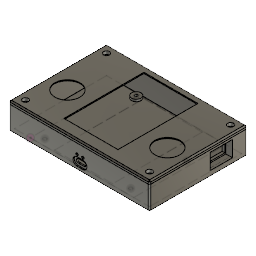
Control-Case (Autodesk Fusion 360 design; units mm, degrees)
Autodesk Fusion 360 part; units mm, degrees
sketch "Skizze1" plane through (0, 0, 0) normal (0, 0, 1) x (1, 0, 0) in component "Case-Bottom"
  line L0 (0, 0) -> (99, 0) construction
  line L1 (99, 0) -> (99, 88) construction
  line L2 (99, 88) -> (0, 88) construction
  line L3 (0, 88) -> (0, 0) construction
  circle A0 centre (7.8, 6.1) radius 1.5 construction
  circle A1 centre (90, 6.1) radius 1.5 construction
  circle A2 centre (94, 55.7) radius 1.5 construction
  circle A3 centre (17.6, 83.8) radius 1.5 construction
  line L4 (21.8, 86.9) -> (77.5, 86.9) construction
  line L5 (77.5, 86.9) -> (77.5, 1.4) construction
  line L6 (77.5, 1.4) -> (21.8, 1.4) construction
  line L7 (21.8, 1.4) -> (21.8, 86.9) construction
  line L8 (-15.1, 0) -> (114.1, 0) construction
  line L9 (114.1, 0) -> (114.1, 88) construction
  line L10 (114.1, 88) -> (-15.1, 88) construction
  line L11 (-15.1, 88) -> (-15.1, 0) construction
  dimension "d1" = 99
  dimension "d2" = 88
  dimension "d3" = 3
  dimension "d4" = 1.4
  dimension "d5" = 86.9
  dimension "d6" = 21.8
  dimension "d7" = 77.5
  dimension "d8" = 7.8
  dimension "d9" = 6.1
  dimension "d10" = 83.8
  dimension "d11" = 17.6
  dimension "d12" = 94
  dimension "d13" = 55.7
  dimension "d14" = 6.1
  dimension "d15" = 90
  dimension "d16" = 15.1
  dimension "d17" = 15.1
  constraint horizontal L0
  constraint vertical L1
  constraint horizontal L2
  constraint vertical L3
  constraint coincident L0.start L3.end
  constraint equal A0 A1
  constraint equal A1 A2
  constraint equal A2 A3
  constraint horizontal L4
  constraint vertical L5
  constraint horizontal L6
  constraint vertical L7
  constraint horizontal L8
  constraint vertical L9
  constraint horizontal L10
  constraint vertical L11
  constraint collinear L2 L10
  constraint collinear L0 L8
  measures "d1" distance of L0.start L0.end
  measures "d2" distance of L0.start L2.end
  measures "d3" diameter of A0
  measures "d4" distance of L0 L6
  measures "d5" distance of L0 L4
  measures "d6" distance of L3 L7
  measures "d7" distance of L3 L5
  measures "d8" distance of L3 A0.centre
  measures "d9" distance of L0 A0.centre
  measures "d10" distance of L0 A3.centre
  measures "d11" distance of L3 A3.centre
  measures "d12" distance of L3 A2.centre
  measures "d13" distance of L0 A2.centre
  measures "d14" distance of L0 A1.centre
  measures "d15" distance of L3 A1.centre
  measures "d16" distance of L3 L11
  measures "d17" distance of L1 L9
sketch "Skizze2" plane through (0, 0, 0) normal (0, 0, 1) x (1, 0, 0) in component "Case-Bottom"
  line L0 (114.1, 0) -> (114.1, 88)
  line L1 (114.1, 88) -> (-15.1, 88)
  line L2 (-15.1, 0) -> (114.1, 0)
  line L3 (-15.1, 88) -> (-15.1, 0)
  line L4 (-15.4, -0.3) -> (114.4, -0.3)
  line L5 (114.4, -0.3) -> (114.4, 88.3)
  line L6 (114.4, 88.3) -> (-15.4, 88.3)
  line L7 (-15.4, 88.3) -> (-15.4, -0.3)
  line L8 (-17.9, 90.8) -> (-17.9, -2.8)
  line L9 (-17.9, -2.8) -> (116.9, -2.8)
  line L10 (116.9, -2.8) -> (116.9, 90.8)
  line L11 (116.9, 90.8) -> (-17.9, 90.8)
  dimension "d18" = 0.3
  dimension "d19" = 2.8
extrude "Extrusion1" add sketch "Skizze2" against normal blind 2 contours L0 L1 L2 L3 | L4 L5 L6 L7 | L8 L9 L10 L11 makes body 1 in component "Case-Bottom"
sketch "Skizze3" plane through (0, 0, 0) normal (0, 0, 1) x (-1, 0, 0) in component "Case-Bottom"
  line L0 (-116.9, -90.8) -> (17.9, -90.8)
  line L1 (17.9, -90.8) -> (17.9, 2.8)
  line L2 (17.9, 2.8) -> (-116.9, 2.8)
  line L3 (-116.9, 2.8) -> (-116.9, -90.8)
  circle A0 centre (-7.8, -6.1) radius 1.5
  circle A1 centre (-17.6, -83.8) radius 1.5
  circle A2 centre (-94, -55.7) radius 1.5
  circle A3 centre (-90, -6.1) radius 1.5
  circle A4 centre (-7.8, -6.1) radius 4.5
  circle A5 centre (-90, -6.1) radius 4.5
  circle A6 centre (-94, -55.7) radius 4.5
  circle A7 centre (-17.6, -83.8) radius 4.5
  circle A8 centre (-7.8, -6.1) radius 1.35
  circle A9 centre (-17.6, -83.8) radius 1.35
  circle A10 centre (-94, -55.7) radius 1.35
  circle A11 centre (-90, -6.1) radius 1.35
  dimension "d22" = 3
  dimension "d23" = 3
  dimension "d25" = 3
  dimension "d26" = 3
  dimension "d113" = 2.7
  constraint concentric A0 A8
  constraint concentric A1 A9
  constraint concentric A2 A10
  constraint concentric A3 A11
  constraint equal A10 A11
  constraint equal A9 A10
  constraint equal A8 A9
  measures "d22" distance of A0
  measures "d23" distance of A3
  measures "d25" distance of A2
  measures "d26" distance of A1
  measures "d113" diameter of A8
extrude "Extrusion2" add sketch "Skizze3" along normal blind 2 contours A0 | A1 | A2 | A3 | A4 | A5 | A6 | A7 bodies 1 in component "Case-Bottom"
extrude "Extrusion3" cut 4 faces at (93.7048, 56.1487, 0) (7.6775, 6.2407, 0) (89.3906, 5.7482, 0) (18.3106, 84.193, 0) along direction (0, 0, -1) blind 1 on bodies 1 bodies 1 in component "Case-Bottom"
sketch "Skizze4" plane through (0, 0, 0) normal (0, 0, 1) x (-1, 0, 0) in component "Case-Bottom"
  circle A0 centre (-17.6, -83.8) radius 4.5
  circle A1 centre (-94, -55.7) radius 4.5
  line L0 (-116.9, -90.8) -> (17.9, -90.8)
  line L1 (17.9, -90.8) -> (17.9, 2.8)
  line L2 (17.9, 2.8) -> (-116.9, 2.8)
  line L3 (-116.9, 2.8) -> (-116.9, -90.8)
  circle A2 centre (-7.8, -6.1) radius 4.5
  circle A3 centre (-90, -6.1) radius 4.5
  line L4 (15.4, -88.3) -> (15.4, 0.3)
  line L5 (15.4, 0.3) -> (-114.4, 0.3)
  line L6 (-114.4, 0.3) -> (-114.4, -88.3)
  line L7 (-114.4, -88.3) -> (15.4, -88.3)
  dimension "d31" = -2.5
extrude "Extrusion4" add sketch "Skizze4" along normal blind 20.8 separate body contours L0 L1 L2 L3 makes body 2 in component "Case-Bottom"
combine "Kombinieren1" operation add target body 1 tool bodies 2 in component "Case-Bottom"
sketch "Skizze1 (2)" plane through (0, 0, 20.8) normal (0, 0, 1) x (-1, 0, 0) in component "Case-Top"
  line L0 (15.4, -88.3) -> (-114.4, -88.3)
  line L1 (-114.4, -88.3) -> (-114.4, 0.3)
  line L2 (15.4, 0.3) -> (15.4, -88.3)
  line L3 (-116.9, 2.8) -> (-116.9, -90.8)
  line L4 (-116.9, -90.8) -> (17.9, -90.8)
  line L5 (17.9, -90.8) -> (17.9, 2.8)
  line L6 (17.9, 2.8) -> (-116.9, 2.8)
  line L7 (17.9, 2.8) -> (-116.9, 2.8)
  line L8 (-116.9, 2.8) -> (-116.9, -90.8)
  line L9 (-116.9, -90.8) -> (17.9, -90.8)
  line L10 (17.9, -90.8) -> (17.9, 2.8)
  line L11 (-21.8, -1.4) -> (-21.8, -86.9)
  line L12 (-77.5, -1.4) -> (-21.8, -1.4)
  line L13 (-77.5, -86.9) -> (-77.5, -1.4)
  line L14 (-21.8, -86.9) -> (-77.5, -86.9)
  line L15 (-23.8, -84.9) -> (-75.5, -84.9)
  line L16 (-75.5, -84.9) -> (-75.5, -8.4)
  line L17 (-75.5, -8.4) -> (-23.8, -8.4)
  line L18 (-23.8, -8.4) -> (-23.8, -84.9)
  circle A0 centre (-1.8, -33.7) radius 12
  circle A1 centre (-97.5, -33.7) radius 12
  line L19 (-114.4, 0.3) -> (15.4, 0.3)
  line L20 (-21.6, -1.2) -> (-21.6, -87.1)
  line L21 (-21.6, -87.1) -> (-77.7, -87.1)
  line L22 (-77.7, -87.1) -> (-77.7, -1.2)
  line L23 (-77.7, -1.2) -> (-21.6, -1.2)
  dimension "d34" = 7
  dimension "d35" = 2
  dimension "d36" = 2
  dimension "d37" = 2
  dimension "d43" = 34
  dimension "d44" = 34
  dimension "d45" = 24
  dimension "d46" = 20
  dimension "d47" = 20
  dimension "d112" = -0.2
  constraint horizontal L7
  constraint vertical L8
  constraint horizontal L9
  constraint vertical L10
  constraint coincident L3.end L4.start
  constraint coincident L5.end L6.start
  constraint horizontal L15
  constraint vertical L16
  constraint horizontal L17
  constraint vertical L18
  constraint equal A0 A1
  measures "d34" distance of L12 L17
  measures "d35" distance of L13 L16
  measures "d36" distance of L14 L15
  measures "d37" distance of L11 L18
  measures "d43" distance of A0.centre L19
  measures "d44" distance of A1.centre L19
  measures "d45" diameter of A0
  measures "d46" distance of L11 A0.centre
  measures "d47" distance of L13 A1.centre
extrude "Extrusion1'" add sketch "Skizze1 (2)" along normal blind 2 separate body contours L0 L1 L2 L19 | L3 L4 L5 L6 L7 L8 L9 L10 | L11 L12 L13 L14 | L20 L21 L22 L23 makes body 3 in component "Case-Top"
extrude "Extrusion2'" cut sketch "Skizze1 (2)" along normal blind 1 contours L11 L12 L13 L14 | L20 L21 L22 L23 bodies 3 in component "Case-Top"
chamfer "Fase1" distance 1.4 angle 45 2 edges at (12.9879, 29.3606, 20.8) (108.6879, 29.3606, 20.8) on bodies 3 in component "Case-Top"
sketch "Skizze2 (2)" plane through (0, 0, 22.8) normal (0, 0, 1) x (-1, 0, 0) in component "Case-Top"
  line L0 (-75.5, -8.4) -> (-23.8, -8.4)
  line L1 (-23.8, -8.4) -> (-23.8, -84.9)
  line L2 (-23.8, -84.9) -> (-75.5, -84.9)
  line L3 (-75.5, -84.9) -> (-75.5, -8.4)
  circle A0 centre (-97.5, -33.7) radius 12
  circle A1 centre (-1.8, -33.7) radius 12
  line L4 (17.9, -90.8) -> (17.9, 2.8)
  line L5 (17.9, 2.8) -> (-116.9, 2.8)
  line L6 (-116.9, 2.8) -> (-116.9, -90.8)
  line L7 (-116.9, -90.8) -> (17.9, -90.8)
  line L8 (-108.9, -82.8) -> (9.9, -82.8) construction
  line L9 (9.9, -82.8) -> (9.9, -5.2) construction
  line L10 (9.9, -5.2) -> (-108.9, -5.2) construction
  line L11 (-108.9, -5.2) -> (-108.9, -82.8) construction
  circle A2 centre (9.9, -5.2) radius 2.8
  circle A3 centre (9.9, -82.8) radius 2.8
  circle A4 centre (-108.9, -82.8) radius 2.8
  circle A5 centre (-108.9, -5.2) radius 2.8
  dimension "d49" = -8
  dimension "d50" = 5.6
  constraint coincident L9.end L10.start
  constraint coincident L8.end L9.start
  constraint coincident L8.start L11.end
  constraint coincident L10.end L11.start
  constraint equal A4 A5
  constraint equal A3 A4
  constraint equal A2 A3
  measures "d50" diameter of A2
extrude "Extrusion3'" cut sketch "Skizze2 (2)" against normal blind 2 contours A2 | A3 | A4 | A5 bodies 3 in component "Case-Top"
sketch "Skizze3 (2)" plane through (0, 0, 20.8) normal (0, 0, -1) x (1, 0, 0) in component "Case-Top"
  circle A0 centre (108.9, -82.8) radius 2.8
  circle A1 centre (108.9, -5.2) radius 2.8
  circle A2 centre (-9.9, -82.8) radius 2.8
  circle A3 centre (-9.9, -5.2) radius 2.8
  circle A4 centre (1.8, -33.7) radius 13.4
  line L0 (-17.9, 2.8) -> (-17.9, -90.8)
  line L1 (-17.9, -90.8) -> (116.9, -90.8)
  line L2 (116.9, -90.8) -> (116.9, 2.8)
  line L3 (116.9, 2.8) -> (-17.9, 2.8)
  circle A5 centre (97.5, -33.7) radius 13.4
  line L4 (-15.4, 0.3) -> (-15.4, -88.3)
  line L5 (-15.4, -88.3) -> (114.4, -88.3)
  line L6 (114.4, -88.3) -> (114.4, 0.3)
  line L7 (114.4, 0.3) -> (-15.4, 0.3)
  circle A6 centre (108.9, -5.2) radius 5
  circle A7 centre (108.9, -82.8) radius 5
  circle A8 centre (-9.9, -82.8) radius 5
  circle A9 centre (-9.9, -5.2) radius 5
  line L8 (21.6, -1.2) -> (77.7, -1.2)
  line L9 (77.7, -1.2) -> (77.7, -87.1)
  line L10 (77.7, -87.1) -> (21.6, -87.1)
  line L11 (21.6, -87.1) -> (21.6, -1.2)
  dimension "d53" = -2.5
  dimension "d54" = 10
  constraint concentric A1 A6
  constraint concentric A0 A7
  constraint concentric A2 A8
  constraint concentric A3 A9
  constraint equal A8 A9
  constraint equal A7 A8
  constraint equal A6 A7
  measures "d54" diameter of A6
extrude "Extrusion4'" add sketch "Skizze3 (2)" along normal blind 1 contours A6 | A7 | A8 | A9 bodies 3 in component "Case-Top"
sketch "Skizze4 (2)" plane through (0, 0, 19.8) normal (0, 0, -1) x (1, 0, 0) in component "Case-Top"
  circle A0 centre (-9.9, -5.2) radius 2.8
  circle A1 centre (-9.9, -5.2) radius 5
  circle A2 centre (-9.9, -5.2) radius 1.45
  circle A3 centre (-9.9, -82.8) radius 5
  circle A4 centre (108.9, -82.8) radius 5
  circle A5 centre (108.9, -5.2) radius 5
  circle A6 centre (-9.9, -82.8) radius 1.45
  circle A7 centre (108.9, -82.8) radius 1.45
  circle A8 centre (108.9, -5.2) radius 1.45
  dimension "d57" = 2.9
  constraint concentric A0 A2
  constraint concentric A3 A6
  constraint concentric A4 A7
  constraint concentric A5 A8
  constraint equal A7 A8
  constraint equal A2 A8
  constraint equal A2 A6
  measures "d57" diameter of A2
extrude "Extrusion5" add sketch "Skizze4 (2)" along normal blind 3 contours A0 | A1 | A3 | A4 | A5 bodies 3 in component "Case-Top"
sketch "Skizze5" plane through (0, 0, 0) normal (0, 0, 1) x (-1, 0, 0) in component "Case-Bottom"
  circle A0 centre (-90, -6.1) radius 4.5
  circle A1 centre (-7.8, -6.1) radius 4.5
  circle A2 centre (-94, -55.7) radius 4.5
  circle A3 centre (-17.6, -83.8) radius 4.5
  line L0 (-17.6, -88.3) -> (15.4, -88.3)
  line L1 (15.4, -88.3) -> (15.4, 0.3)
  line L2 (15.4, 0.3) -> (-114.4, 0.3)
  line L3 (-114.4, 0.3) -> (-114.4, -88.3)
  line L4 (-114.4, -88.3) -> (-17.6, -88.3)
  circle A4 centre (9.9, -5.2) radius 5 construction
  circle A5 centre (-108.9, -5.2) radius 5 construction
  circle A6 centre (-108.9, -82.8) radius 5 construction
  circle A7 centre (9.9, -82.8) radius 5 construction
  line L5 (15.4, -88.3) -> (4.9, -88.3)
  line L6 (4.9, -88.3) -> (4.9, -77.8)
  line L7 (4.9, -77.8) -> (15.4, -77.8)
  line L8 (15.4, -77.8) -> (15.4, -88.3)
  line L9 (15.4, 0.3) -> (4.9, 0.3)
  line L10 (4.9, 0.3) -> (4.9, -10.2)
  line L11 (4.9, -10.2) -> (15.4, -10.2)
  line L12 (15.4, -10.2) -> (15.4, 0.3)
  line L13 (-114.4, -88.3) -> (-103.9, -88.3)
  line L14 (-103.9, -88.3) -> (-103.9, -77.8)
  line L15 (-103.9, -77.8) -> (-114.4, -77.8)
  line L16 (-114.4, -77.8) -> (-114.4, -88.3)
  line L17 (-114.4, 0.3) -> (-103.9, 0.3)
  line L18 (-103.9, 0.3) -> (-103.9, -10.2)
  line L19 (-103.9, -10.2) -> (-114.4, -10.2)
  line L20 (-114.4, -10.2) -> (-114.4, 0.3)
  circle A8 centre (9.9, -82.8) radius 1.35
  circle A9 centre (9.9, -5.2) radius 1.35
  circle A10 centre (-108.9, -5.2) radius 1.35
  circle A11 centre (-108.9, -82.8) radius 1.35
  dimension "d63" = 10.5
  dimension "d64" = 10.5
  dimension "d65" = 10.5
  dimension "d66" = 10.5
  dimension "d67" = 10.5
  dimension "d68" = 10.5
  dimension "d69" = 10.5
  dimension "d70" = 10.5
  dimension "d71" = 2.7
  constraint horizontal L5
  constraint vertical L6
  constraint horizontal L7
  constraint vertical L8
  constraint coincident L0.end L1.start
  constraint horizontal L9
  constraint vertical L10
  constraint horizontal L11
  constraint vertical L12
  constraint coincident L1.end L2.start
  constraint horizontal L13
  constraint vertical L14
  constraint horizontal L15
  constraint vertical L16
  constraint coincident L3.end L4.start
  constraint horizontal L17
  constraint vertical L18
  constraint horizontal L19
  constraint vertical L20
  constraint coincident L2.end L3.start
  constraint concentric A7 A8
  constraint concentric A4 A9
  constraint concentric A5 A10
  constraint concentric A6 A11
  constraint equal A10 A11
  constraint equal A9 A10
  constraint equal A8 A9
  measures "d63" distance of L0.end L5.end
  measures "d64" distance of L0.end L7.end
  measures "d65" distance of L1.end L11.end
  measures "d66" distance of L1.end L9.end
  measures "d67" distance of L3.end L13.end
  measures "d68" distance of L3.end L15.end
  measures "d69" distance of L2.end L19.end
  measures "d70" distance of L2.end L17.end
  measures "d71" diameter of A8
extrude "Extrusion5'" add sketch "Skizze5" along normal blind 17.8 separate body contours L0 L1 L5 L6 L7 L8 | L3 L4 L13 L14 L15 L16 | L1 L2 L9 L10 L11 L12 | L2 L3 L17 L18 L19 L20 makes body 4 at (-8.4, 77.8, 5.9333) makes body 5 at (107.4, 77.8, 5.9333) makes body 6 at (-15.4, 6.7, 5.9333) makes body 7 at (107.4, 10.2, 5.9333) in component "Case-Bottom"
sketch "Skizze6" plane through (0, 77.8, 0) normal (0, -1, 0) x (1, 0, 0) in component "Case-Bottom"
  line L0 (-15.4, 0) -> (-4.9, 0)
  line L1 (-4.9, 0) -> (-4.9, 17.8)
  line L2 (-4.9, 17.8) -> (-15.4, 17.8)
  line L3 (-15.4, 17.8) -> (-15.4, 0)
  line L4 (103.9, 0) -> (114.4, 0)
  line L5 (114.4, 0) -> (114.4, 17.8)
  line L6 (114.4, 17.8) -> (103.9, 17.8)
  line L7 (103.9, 17.8) -> (103.9, 0)
  line L8 (-15.4, 5.3) -> (-4.9, 15.8)
  line L9 (-15.4, 5.3) -> (-0.5508, 5.3) construction
  line L10 (103.9, 15.8) -> (114.4, 5.3)
  line L11 (103.9, 15.8) -> (118.7492, 15.8) construction
  dimension "d74" = 45
  dimension "d75" = 2
  dimension "d76" = 45
  dimension "d77" = 2
  constraint horizontal L9
  constraint coincident L3 L8.start
  constraint coincident L1 L8.end
  constraint horizontal L11
  constraint coincident L7 L10.start
  constraint coincident L5 L10.end
  measures "d74" angle of L8 L9
  measures "d75" distance of L1.end L8.end
  measures "d76" angle of L10 L11
  measures "d77" distance of L6.end L10.start
extrude "Extrusion6" cut sketch "Skizze6" against normal blind 10.5 contours L0 L1 L3 L8 | L4 L5 L7 L10 bodies 4 5 in component "Case-Bottom"
sketch "Skizze7" plane through (0, 10.2, 0) normal (0, 1, 0) x (-1, 0, 0) in component "Case-Bottom"
  line L0 (-114.4, 0) -> (-103.9, 0)
  line L1 (-103.9, 0) -> (-103.9, 17.8)
  line L2 (-103.9, 17.8) -> (-114.4, 17.8)
  line L3 (-114.4, 17.8) -> (-114.4, 0)
  line L4 (4.9, 0) -> (15.4, 0)
  line L5 (15.4, 0) -> (15.4, 17.8)
  line L6 (15.4, 17.8) -> (4.9, 17.8)
  line L7 (4.9, 17.8) -> (4.9, 0)
  line L8 (-103.9, 15.8) -> (-114.4, 5.3)
  line L9 (15.4, 5.3) -> (4.9, 15.8)
extrude "Extrusion7" cut sketch "Skizze7" against normal blind 10.5 contours L0 L1 L3 L8 | L4 L5 L7 L9 bodies 6 7 in component "Case-Bottom"
sketch "Skizze8" plane through (116.9, 0, 0) normal (1, 0, 0) x (0, 1, 0) in component "Case-Bottom"
  line L0 (-2.8, 20.8) -> (-2.8, -2)
  line L1 (-2.8, -2) -> (90.8, -2)
  line L2 (90.8, -2) -> (90.8, 20.8)
  line L3 (90.8, 20.8) -> (-2.8, 20.8)
  line L4 (56.25, 17.5) -> (75.75, 17.5)
  line L5 (75.75, 17.5) -> (75.75, 4.9)
  line L6 (75.75, 4.9) -> (56.25, 4.9)
  line L7 (56.25, 4.9) -> (56.25, 17.5)
  line L8 (56.25, 11.2) -> (75.75, 11.2) construction
  line L9 (76.6, 18.8) -> (55.4, 18.8)
  line L10 (55.4, 18.8) -> (55.4, 3.6)
  line L11 (55.4, 3.6) -> (76.6, 3.6)
  line L12 (76.6, 3.6) -> (76.6, 18.8)
  line L13 (76.6, 18.8) -> (55.4, 3.6) construction
  line L14 (55.4, 18.8) -> (76.6, 3.6) construction
  line L15 (77.8, 5.3) -> (77.8, 17.8) construction
  line L16 (88.3, 20.8) -> (-0.3, 20.8) construction
  point P0 (66, 11.2)
  dimension "d82" = 19.5
  dimension "d83" = 12.6
  dimension "d84" = 21.2
  dimension "d85" = 15.2
  dimension "d86" = 1.2
  dimension "d87" = 2
  constraint horizontal L4
  constraint vertical L5
  constraint horizontal L6
  constraint vertical L7
  constraint midpoint L7 L8.start
  constraint midpoint L5 L8.end
  constraint perpendicular L9 L10
  constraint parallel L9 L11
  constraint parallel L10 L12
  constraint horizontal L9
  constraint coincident L13 P0
  constraint coincident L14 P0
  constraint midpoint L8 P0
  measures "d82" distance of L4.start L4.end
  measures "d83" distance of L4.start L6.end
  measures "d84" distance of L10.end L11.end
  measures "d85" distance of L9.end L10.end
  measures "d86" distance of L12 L15
  measures "d87" distance of L9 L16
extrude "Extrusion8" cut sketch "Skizze8" against normal blind 2.5 contours L4 L5 L6 L7 bodies 1 in component "Case-Bottom"
sketch "Skizze9" plane through (114.4, 0, 0) normal (-1, 0, 0) x (0, -1, 0) in component "Case-Bottom"
  line L0 (-75.75, 4.9) -> (-75.75, 17.5)
  line L1 (-75.75, 17.5) -> (-56.25, 17.5)
  line L2 (-56.25, 17.5) -> (-56.25, 4.9)
  line L3 (-56.25, 4.9) -> (-75.75, 4.9)
  line L4 (0.3, 0) -> (0.3, 20.8)
  line L5 (0.3, 20.8) -> (-88.3, 20.8)
  line L6 (-88.3, 20.8) -> (-88.3, 0)
  line L7 (-77.75, 2.9) -> (-77.75, 19.5)
  line L8 (-77.75, 19.5) -> (-54.25, 19.5)
  line L9 (-54.25, 19.5) -> (-54.25, 2.9)
  line L10 (-54.25, 2.9) -> (-77.75, 2.9)
  line L11 (-88.3, 0) -> (0.3, 0)
  dimension "d90" = -2
extrude "Extrusion9" add sketch "Skizze9" along normal blind 6.5 separate body contours L7 L8 L9 L10 makes body 8 in component "Case-Bottom"
extrude "Extrusion10" cut sketch "Skizze8" against normal blind 6.4 contours L9 L10 L11 L12 bodies 1 8 in component "Case-Bottom"
combine "Kombinieren2" operation add target body 1 tool bodies 7 6 8 4 5 in component "Case-Bottom"
sketch "Skizze10" plane through (0, -2.8, 0) normal (0, -1, 0) x (1, 0, 0) in component "Case-Bottom"
  line L0 (-17.9, 20.8) -> (-17.9, -2)
  line L1 (-17.9, -2) -> (116.9, -2)
  line L2 (116.9, -2) -> (116.9, 20.8)
  line L3 (116.9, 20.8) -> (-17.9, 20.8)
  line L4 (47.5, 3.6) -> (53.1, 3.6)
  arc A0 (53.1, 3.6) -> (53.1, 7.4) centre (53.1, 5.5) ccw
  line L5 (53.1, 7.4) -> (47.5, 7.4)
  arc A1 (47.5, 7.4) -> (47.5, 3.6) centre (47.5, 5.5) ccw
  line L6 (47.5, 5.5) -> (53.1, 5.5) construction
  line L7 (98.5, 2) -> (89.5, 2)
  line L8 (47.5, 5.5) -> (47.5, 11.5) construction
  circle A2 centre (47.5, 11.5) radius 1.25
  line L9 (53.1, 5.5) -> (53.1, 11.5) construction
  circle A3 centre (53.1, 11.5) radius 1.25
  line L10 (92.65, 2) -> (95.35, 2)
  point P0 (99, 0)
  dimension "d95" = 3.8
  dimension "d96" = 5.6
  dimension "d97" = 45.9
  dimension "d98" = 1.6
  dimension "d104" = 6
  dimension "d105" = 2.5
  dimension "d106" = 2.5
  constraint tangent L4 A0
  constraint tangent A0 L5
  constraint parallel L4 L5
  constraint tangent L5 A1
  constraint tangent L4 A1
  constraint parallel L3 L6
  constraint coincident A1.centre L6.start
  constraint perpendicular L6 L8
  constraint coincident L8.end A2.centre
  constraint coincident A0.centre L6.end
  constraint perpendicular L6 L9
  constraint coincident L9.end A3.centre
  measures "d95" distance of L4 L5
  measures "d96" distance of A1.centre A0.centre
  measures "d97" horizontal distance of A0.centre P0
  measures "d98" distance of L4 L7
  measures "d104" distance of A1.centre L8.end
  measures "d105" diameter of A2
  measures "d106" diameter of A3
extrude "Extrusion13" cut sketch "Skizze10" against normal blind 2.5 contours A2 | A3 bodies 1 in component "Case-Bottom"
extrude "Extrusion11" cut sketch "Skizze10" against normal blind 2.5 contours L4 A0 L5 A1 bodies 1 in component "Case-Bottom"
sketch "Skizze11" plane through (0, -2.8, 0) normal (0, -1, 0) x (1, 0, 0) in component "Case-Bottom"
  line L0 (53.1, 3.6) -> (47.5, 3.6)
  arc A0 (47.5, 7.4) -> (47.5, 3.6) centre (47.5, 5.5) ccw
  line L1 (47.5, 7.4) -> (53.1, 7.4)
  arc A1 (53.1, 3.6) -> (53.1, 7.4) centre (53.1, 5.5) ccw
  line L2 (-17.9, 20.8) -> (-17.9, -2)
  line L3 (116.9, -2) -> (116.9, 20.8)
  line L4 (116.9, 20.8) -> (-17.9, 20.8)
  arc A2 (47.5, 9.4) -> (47.5, 1.6) centre (47.5, 5.5) ccw
  line L5 (53.1, 1.6) -> (47.5, 1.6)
  arc A3 (53.1, 1.6) -> (53.1, 9.4) centre (53.1, 5.5) ccw
  line L6 (47.5, 9.4) -> (53.1, 9.4)
  circle A4 centre (47.5, 11.5) radius 1.25
  circle A5 centre (53.1, 11.5) radius 1.25
  line L7 (-17.9, -2) -> (116.9, -2)
  dimension "d101" = -2
extrude "Extrusion12" cut sketch "Skizze11" against normal blind 1.2 contours A2 L5 A3 L6 bodies 1 in component "Case-Bottom"
chamfer "Fase1'" distance 1.5 angle 45 2 edges at (51.9346, -0.3, 11.048) (46.3346, -0.3, 11.048) on bodies 1 in component "Case-Bottom"
chamfer "Fase2" distance 1.2 angle 45 8 edges at (-17.9, -2.8, 9.4) (-17.9, 44, -2) (49.5, -2.8, -2) (-17.9, 90.8, 9.4) (49.5, 90.8, -2) (116.9, 90.8, 9.4) (116.9, 44, -2) (116.9, -2.8, 9.4) on bodies 1 in component "Case-Bottom"
chamfer "Fase2'" distance 1.2 angle 45 8 edges at (-17.9, -2.8, 21.8) (49.5, -2.8, 22.8) (-17.9, 44, 22.8) (49.5, 90.8, 22.8) (-17.9, 90.8, 21.8) (116.9, 90.8, 21.8) (116.9, 44, 22.8) (116.9, -2.8, 21.8) on bodies 3 in component "Case-Top"
sketch "Skizze1 (3)" plane through (0, 0, 21.8) normal (0, 0, -1) x (1, 0, 0)
  line L0 (115.7, -90.8) -> (116.9, -89.6)
  line L1 (116.9, -89.6) -> (116.9, 1.6)
  line L2 (116.9, 1.6) -> (115.7, 2.8)
  line L3 (115.7, 2.8) -> (-16.7, 2.8)
  line L4 (-16.7, 2.8) -> (-17.9, 1.6)
  line L5 (-17.9, 1.6) -> (-17.9, -89.6)
  line L6 (-17.9, -89.6) -> (-16.7, -90.8)
  line L7 (-16.7, -90.8) -> (115.7, -90.8)
  circle A0 centre (-9.9, -5.2) radius 5
  circle A1 centre (-9.9, -82.8) radius 5
  circle A2 centre (108.9, -5.2) radius 5
  circle A3 centre (108.9, -82.8) radius 5
  circle A4 centre (1.8, -33.7) radius 13.4
  line L8 (21.6, -1.2) -> (77.7, -1.2)
  line L9 (77.7, -1.2) -> (77.7, -87.1)
  line L10 (77.7, -87.1) -> (21.6, -87.1)
  line L11 (21.6, -87.1) -> (21.6, -1.2)
  circle A5 centre (97.5, -33.7) radius 13.4
  line L12 (-15.4, 0.3) -> (-15.4, -88.3)
  line L13 (-15.4, -88.3) -> (114.4, -88.3)
  line L14 (114.4, -88.3) -> (114.4, 0.3)
  line L15 (114.4, 0.3) -> (-15.4, 0.3)
  dimension "d114" = -2.5
extrude "Extrusion6'" add sketch "Skizze1 (3)" along normal blind 1 contours L0 L1 L2 L3 L4 L5 L6 L7 sketch seen with x (1, 0, 0) y (0, 1, 0) z (0, 0, 1) at (0, 0, -1) bodies 3 in component "Case-Top"
component "Case-Bottom" placed x (1, 0, 0) y (0, 1, 0) z (0, 0, 1) at (0, 0, 0)
component "Case-Top" placed x (1, 0, 0) y (0, 1, 0) z (0, 0, 1) at (0, 0, 1)
equation "d19 = 2.5 mm + 0.3 mm"
equation "d32 = 2.00 mm + 19.8 mm - 1 mm"
equation "d35 = d36"
equation "d37 = d36"
equation "d91 = 2.6 mm + 6.4 mm - 2.5 mm"
equation "d96 = 9.4 mm - 3.8 mm"
equation "d97 = 44 mm + 1.9 mm"
